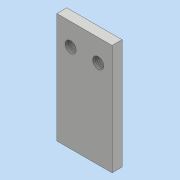
# Autodesk Inventor part: P10
Saved by Autodesk Inventor 2017 (Build 210142000, 142)
## iProperties
Part Number: P10
Material: 一般
Document SubType Name: Modeling
Designer: d8910
Density: 1 g/cm^3
Appearance: 預設
Author: d8910
Autodesk Inventor part; units mm, degrees
ref_plane "YZ Plane" through (0, 0, 0) normal (1, 0, 0) x (0, 1, 0)
ref_plane "XZ Plane" through (0, 0, 0) normal (0, 1, 0) x (-1, 0, 0)
ref_plane "XY Plane" through (0, 0, 0) normal (0, 0, 1) x (1, 0, 0)
sketch "草圖1" plane through (0, 0, 0) normal (0, 1, 0) x (-1, 0, 0)
  line L0 (25, 50) -> (-25, 50)
  line L1 (-25, 50) -> (-25, -50)
  line L2 (-25, -50) -> (25, -50)
  line L3 (25, -50) -> (25, 50)
  circle A0 centre (12.5, 30) radius 5
  circle A1 centre (-12.5, 30) radius 5
  point P0 (0, 0)
  point P1 (25, 0)
  point P2 (0, -50)
  dimension "d0" = 50
  dimension "d1" = 100
  dimension "d2" = 25
  dimension "d3" = 12.5
  dimension "d4" = 10
  dimension "d5" = 20
  constraints: 8 end point, 2 centre point, 2 horizontal alignment, 2 midpoint, 2 parallel, 1 equal radius, 1 horizontal, 1 perpendicular, 1 vertical alignment
  measures "d0" distance of L1.end L2.end
  measures "d1" distance of L0.end L1.end
  measures "d2" distance of A0.centre A1.centre
  measures "d3" horizontal distance of point (0, 0) A1.centre
  measures "d4" diameter of A0
  measures "d5" distance from line of L0 A1.centre
extrude "擠出1" add sketch "草圖1" along normal blind 10
chamfer "倒角1" distance 1 angle 45 4 edges at (0, 10, 50) (-25, 10, 0) (25, 10, 0) (0, 10, -50)
thread "螺紋1" size "M10x1.25" class "6H" standard "ISO Metric profile" full length
thread "螺紋2" size "M10x1.5" class "6H" standard "ANSI Metric M Profile" full length
